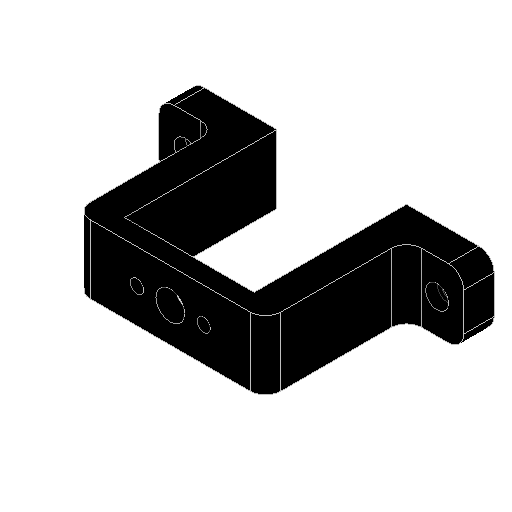
# Autodesk Inventor part: Motor _Fixation
Saved by Autodesk Inventor 2025.2 (Build 292293000, 293)
## iProperties
Created: 2025-12-09
Part Number: Motor _Fixation
Material: Generic
Document SubType Name: Modeling
Designer: Access
Density: 1 g/cm^3
Appearance: Anodized - Black
Author: Access
Autodesk Inventor part; units mm, degrees
ref_plane "YZ Plane" through (0, 0, 0) normal (1, 0, 0) x (0, 1, 0)
ref_plane "XZ Plane" through (0, 0, 0) normal (0, 1, 0) x (-1, 0, 0)
ref_plane "XY Plane" through (0, 0, 0) normal (0, 0, 1) x (1, 0, 0)
sketch "Sketch1" plane through (0, 0, 0) normal (0, 0, 1) x (1, 0, 0)
  circle A0 centre (0, 0) radius 3.75
  circle A1 centre (-8.75, 0) radius 1.75
  line L0 (-35, 0) -> (35, 0) projected
  line L1 (0, 0) -> (0, 3.75)
  circle A2 centre (8.75, 0) radius 1.75
  line L2 (-25, 9) -> (25, 9)
  line L3 (25, 9) -> (25, -9)
  line L4 (25, -9) -> (-25, -9)
  line L5 (-25, -9) -> (-25, 9)
  line L6 (0, -12.6) -> (0, 12.6) projected
  line L7 (25, 9) -> (17, 9)
  line L8 (17, 9) -> (17, -9)
  line L9 (17, -9) -> (25, -9)
  line L10 (25, -9) -> (25, 9)
  line L11 (-25, 9) -> (-25, -9)
  line L12 (-25, 9) -> (-17, 9)
  line L13 (-17, 9) -> (-17, -9)
  line L14 (-17, -9) -> (-25, -9)
  point P0 (0, 9)
  point P1 (25, 0)
  point P2 (-17, -9)
  point P3 (17, 9)
  point P4 (-17, 9)
  dimension "d2" = 7.5
  dimension "d3" = 3.5
  dimension "d4" = 8.75
  dimension "d5" = 18
  dimension "d6" = 50
  dimension "d9" = 8
  constraints: 26 end point, 5 symmetric about line, 4 parallel, 4 point on line, 2 centre point, 2 horizontal, 2 midpoint, 2 perpendicular, 1 coincident, 1 vertical, 1 vertical alignment, 3 other
  measures "d3" diameter of A1
  measures "d4" distance of A1.centre point (0, 0)
  measures "d5" distance of L2.end L3.end
  measures "d6" distance of L3.end L4.end
  measures "d9" distance of L9.end L8.end
extrude "Extrusion1" add sketch "Sketch1" against normal blind 5 contours L0 A2 L8 L4 L6 A0 | A0 L6 L2 L8 L0 A2 | A0 L0 A1 L13 L2 L6 | L6 L4 L13 L0 A1 A0
extrude "Extrusion2" add sketch "Sketch1" against normal blind 45 contours L13 L0 L5 L2 | L2 L3 L0 L8 | L8 L0 L3 L4 | L4 L5 L0 L13
sketch "Sketch2" plane through (25, -9, 0) normal (1, 0, 0) x (0, 0, -1)
  line L0 (5, 0) -> (45, 0) projected
  line L1 (37, 0) -> (45, 0)
  line L2 (45, 0) -> (45, 18)
  line L3 (45, 18) -> (37, 18)
  line L4 (37, 18) -> (37, 0)
  point P0 (0, 9)
  dimension "d12" = 8
  constraints: 8 end point, 2 parallel, 1 horizontal, 1 perpendicular, 1 point on line
  measures "d12" distance of L2.end L3.end
extrude "Extrusion3" add sketch "Sketch2" along normal blind 15
sketch "Sketch3" plane through (25, -9, -37) normal (0, 0, 1) x (1, 0, 0)
  circle A0 centre (8, 9) radius 1.75
  line L0 (-63, 9) -> (28, 9) projected
  line L1 (0, 0) -> (0, 18) projected
  point P0 (-25, 9)
  dimension "d15" = 3.5
  dimension "d16" = 8
  constraints: 1 centre point, 1 point on line
  measures "d15" diameter of A0
  measures "d16" distance from line of A0.centre L1
extrude "Extrusion4" cut sketch "Sketch3" against normal blind 15
mirror "Mirror1" about plane through (0, 0, 0) normal (1, 0, 0) of "Extrusion3", "Extrusion4"
sketch "Sketch4" plane through (0, 0, -45) normal (0, 0, -1) x (-1, 0, 0)
  point P0 (0, 0)
sketch "Sketch5" plane through (25, -9, -37) normal (0, 0, 1) x (1, 0, 0)
  circle A0 centre (8, 9) radius 1.75 projected
  circle A1 centre (8, 9) radius 3
  circle A2 centre (-33.75, 9) radius 1.75 projected
  circle A3 centre (-58, 9) radius 1.75 projected
  circle A4 centre (-58, 9) radius 3
  point P0 (-25, 9)
  dimension "d19" = 6
  constraints: 2 centre point, 2 coincident, 1 equal radius
  measures "d19" diameter of A1
extrude "Extrusion5" cut sketch "Sketch5" against normal blind 3 contours A1 | A4
fillet "Fillet1" radius 4 8 edges at (25, 0, -37) (25, 0, 0) (-25, 0, 0) (-25, 0, -37) (-40, -9, -41) (-40, 9, -41) (40, -9, -41) (40, 9, -41)
body "Solid1"
